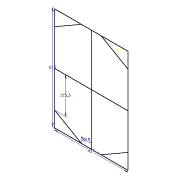
# Autodesk Inventor part: mount_holes_plate
Saved by Autodesk Inventor 2014 SP1 (Build 180222100, 222)
## iProperties
Created: 2015-02-04
Part Number: mount_holes_plate
Material: Generic
Document SubType Name: Modeling
Designer: Simen
Density: 1 g/cm^3
Appearance: Default
Author: Simen
Autodesk Inventor part; units mm, degrees
ref_plane "YZ Plane" through (0, 0, 0) normal (1, 0, 0) x (0, 1, 0)
ref_plane "XZ Plane" through (0, 0, 0) normal (0, 1, 0) x (-1, 0, 0)
ref_plane "XY Plane" through (0, 0, 0) normal (0, 0, 1) x (1, 0, 0)
sketch "Sketch1" plane through (0, 0, 0) normal (0, 1, 0) x (-1, 0, 0)
  line L0 (75.2406, 23.4715) -> (252.2406, 23.4715)
  line L1 (382.2406, -68.5285) -> (382.2406, -499.5285)
  line L2 (252.2406, -591.5285) -> (75.2406, -591.5285)
  line L3 (-54.7594, -499.5285) -> (-54.7594, -68.5285)
  line L4 (-54.7594, -284.0285) -> (382.2406, -284.0285)
  line L5 (382.2406, -284.0285) -> (382.2406, -499.5285)
  line L6 (163.7406, 23.4715) -> (163.7406, -591.5285)
  line L7 (163.7406, -591.5285) -> (252.2406, -591.5285)
  line L8 (252.2406, -591.5285) -> (382.2406, -499.5285)
  line L9 (75.2406, -591.5285) -> (-54.7594, -499.5285)
  line L10 (252.2406, 23.4715) -> (382.2406, -68.5285)
  line L11 (75.2406, 23.4715) -> (-54.7594, -68.5285)
  point P0 (0, 0)
  dimension "d0" = 437
  dimension "d2" = 215.5
  dimension "d3" = 88.5
  dimension "d4" = 615
  constraints: 24 end point, 6 symmetric about line, 4 midpoint, 2 parallel, 1 horizontal, 1 perpendicular
  measures "d0" distance of L1.end L3.start
  measures "d2" distance of L1.end L4.end
  measures "d3" distance of L2.start L6.end
  measures "d4" distance of L6.start L6.end
extrude "Extrusion1" add sketch "Sketch1" along normal blind 10
sketch "Sketch2" plane through (0, 10, 0) normal (0, 1, 0) x (1, 0, 0)
  line L0 (-382.2406, 499.5285) -> (-382.2406, 68.5285) projected
  line L1 (-252.2406, -23.4715) -> (-75.2406, -23.4715) projected
  line L2 (-75.2406, -23.4715) -> (54.7594, 68.5285) projected
  line L3 (54.7594, 68.5285) -> (54.7594, 499.5285) projected
  line L4 (54.7594, 499.5285) -> (-75.2406, 591.5285) projected
  line L5 (-75.2406, 591.5285) -> (-252.2406, 591.5285) projected
  line L6 (-163.7406, 591.5285) -> (-163.7406, -23.4715)
  line L7 (-382.2406, 499.5285) -> (54.7594, 499.5285)
  line L8 (-163.7406, 499.5285) -> (-90.7406, 499.5285)
  line L9 (-90.7406, 499.5285) -> (39.2594, 499.5285)
  line L10 (39.2594, 499.5285) -> (39.2594, 510.4977)
  line L11 (-382.2406, 284.0285) -> (54.7594, 284.0285)
  circle A0 centre (39.2594, 284.0285) radius 2.5
  line L12 (39.2594, 284.0285) -> (39.2594, 357.0285)
  line L13 (39.2594, 359.5285) -> (39.2594, 430.0285)
  circle A1 centre (39.2594, 357.0285) radius 2.5
  circle A2 centre (39.2594, 211.0285) radius 2.5
  circle A3 centre (-366.7406, 357.0285) radius 2.5
  circle A4 centre (-366.7406, 211.0285) radius 2.5
  line L14 (39.2594, 393.5285) -> (-90.7406, 393.5285)
  line L15 (-90.7406, 393.5285) -> (-90.7406, 540.5285)
  circle A5 centre (39.2594, 430.0285) radius 2.5
  line L16 (-90.7406, 430.0285) -> (-90.7406, 576.0285)
  circle A6 centre (-90.7406, 576.0285) radius 2.5
  line L17 (-382.2406, 68.5285) -> (54.7594, 68.5285)
  circle A7 centre (39.2594, 138.0285) radius 2.5
  circle A8 centre (-90.7406, -7.9715) radius 2.5
  circle A9 centre (-366.7406, 430.0285) radius 2.5
  circle A10 centre (-236.7406, 576.0285) radius 2.5
  circle A11 centre (-236.7406, -7.9715) radius 2.5
  circle A12 centre (-366.7406, 138.0285) radius 2.5
  line L18 (-90.7406, 499.5285) -> (-90.7406, 68.5285)
  line L19 (-90.7406, -23.4715) -> (-90.7406, -34.4408)
  line L20 (-90.7406, 499.5285) -> (-90.7406, 573.5285)
  line L21 (-90.7406, 591.5285) -> (-90.7406, 602.4977)
  line L22 (39.2594, 499.5285) -> (39.2594, 281.5285)
  line L23 (39.2594, 68.5285) -> (39.2594, 57.5592)
  circle A13 centre (-366.7406, 284.0285) radius 2.5
  point P0 (0, 0)
  dimension "d9" = 5
  dimension "d12" = 5
  dimension "d22" = 5
  dimension "d7" = 73
  dimension "d8" = 130
  dimension "d10" = 73
  dimension "d11" = 73
  dimension "d19" = 5
  dimension "d20" = 615
  dimension "d21" = 146
  dimension "d23" = 437
  dimension "d25" = 5
  constraints: 36 end point, 19 point on line, 11 centre point, 9 symmetric about line, 7 perpendicular, 6 collinear, 5 midpoint, 3 coincident, 3 vertical alignment, 15 other
  measures "d7" distance of L8.start L8.end
  measures "d8" distance of L8.end L9.end
  measures "d10" distance of L12.start L12.end
  measures "d11" distance of L12.end L13.end
  measures "d19" diameter of A5
  measures "d20" distance of L6.start L6.end
  measures "d21" distance of L16.start L16.end
  measures "d23" distance of L0.end L2.end
  measures "d25" diameter of A13
extrude "Extrusion2" cut sketch "Sketch2" against normal blind 10 contours A6 | A13 L11 | L11 A13 | A0 L12 L11 | L11 L22 A0 | L22 L13 A5 | A5 L13 L22 | L12 A0 L11 | L11 A0 L22 | A1 L22 L12 | L12 L22 A1 | A2 | A3 | A4 | A7 | A8 | A9 | A10 | A11 | A12
sketch "Sketch3" plane through (0, 10, 0) normal (0, 1, 0) x (1, 0, 0)
  line L0 (-382.2406, 499.5285) -> (-382.2406, 68.5285) projected
  line L1 (-382.2406, 68.5285) -> (-252.2406, -23.4715) projected
  line L2 (-252.2406, -23.4715) -> (-75.2406, -23.4715) projected
  line L3 (-75.2406, -23.4715) -> (54.7594, 68.5285) projected
  line L4 (54.7594, 68.5285) -> (54.7594, 499.5285) projected
  line L5 (54.7594, 499.5285) -> (-75.2406, 591.5285) projected
  line L6 (-75.2406, 591.5285) -> (-252.2406, 591.5285) projected
  line L7 (-252.2406, 591.5285) -> (-382.2406, 499.5285) projected
  line L8 (-85.1002, 560.5285) -> (23.7594, 483.4894)
  line L9 (23.7594, 483.4894) -> (23.7594, 84.5676)
  line L10 (23.7594, 84.5676) -> (-85.1002, 7.5285)
  line L11 (-85.1002, 7.5285) -> (-242.381, 7.5285)
  line L12 (-242.381, 7.5285) -> (-351.2406, 84.5676)
  line L13 (-351.2406, 84.5676) -> (-351.2406, 483.4894)
  line L14 (-351.2406, 483.4894) -> (-242.381, 560.5285)
  line L15 (-242.381, 560.5285) -> (-85.1002, 560.5285)
  line L16 (-382.2406, 319.1066) -> (-351.2406, 319.1066)
  point P0 (0, 0)
  dimension "d26" = 31
  constraints: 18 end point, 2 point on line, 1 perpendicular, 7 other
  measures "d26" distance of L16.start L16.end
extrude "Extrusion3" cut sketch "Sketch3" against normal blind 10 contours L13 L14 L15 L8 L9 L10 L11 L12
body "Solid1"
